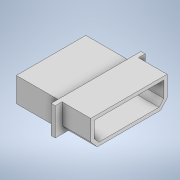
# Autodesk Inventor part: MolexConnector
Saved by Autodesk Inventor 2021 (Build 250183000, 183)
## iProperties
Created: 2021-02-27
Part Number: MolexConnector
Material: Generic
Document SubType Name: Modeling
Designer: Collin
Density: 1 g/cm^3
Appearance: Default
Author: Collin
Autodesk Inventor part; units mm, degrees
ref_plane "YZ Plane" through (0, 0, 0) normal (1, 0, 0) x (0, 1, 0)
ref_plane "XZ Plane" through (0, 0, 0) normal (0, 1, 0) x (-1, 0, 0)
ref_plane "XY Plane" through (0, 0, 0) normal (0, 0, 1) x (1, 0, 0)
sketch "Sketch1" plane through (0, 0, 0) normal (0, 1, 0) x (-1, 0, 0)
  line L0 (-11.8618, -11.6459) -> (11.8618, -11.6459)
  line L1 (11.8618, -11.6459) -> (11.8618, 11.6459)
  line L2 (11.8618, 11.6459) -> (-11.8618, 11.6459)
  line L3 (-11.8618, 11.6459) -> (-11.8618, -11.6459)
  line L4 (-11.8618, -11.6459) -> (11.8618, 11.6459) construction
  line L5 (11.8618, -11.6459) -> (-11.8618, 11.6459) construction
  point P0 (0, 0)
  dimension "d0" = 23.2918
  dimension "d1" = 23.7236
  constraints: 12 end point, 2 midpoint, 2 parallel, 1 horizontal, 1 perpendicular
  measures "d0" distance between parallel lines of L0 L2
  measures "d1" distance of L1.end L2.end
extrude "Extrusion1" add sketch "Sketch1" along normal mid plane 8.509
sketch "Sketch2" plane through (0, 4.2545, 0) normal (0, 1, 0) x (1, 0, 0)
  line L0 (-11.8618, 11.6459) -> (-11.8618, -11.6459) projected
  line L1 (11.8618, 11.6459) -> (-11.8618, 11.6459) projected
  line L2 (-11.8618, -11.6459) -> (1.8542, -11.6459)
  line L3 (1.8542, -11.6459) -> (1.8542, 11.6459)
  line L4 (1.8542, 11.6459) -> (-11.8618, 11.6459)
  line L5 (-11.8618, 11.6459) -> (-11.8618, -11.6459)
  point P0 (0, 0)
  dimension "d4" = 13.716
  constraints: 8 end point, 2 parallel, 1 horizontal, 1 perpendicular, 1 point on line
  measures "d4" distance between parallel lines of L3 L0
extrude "Extrusion2" cut sketch "Sketch2" against normal blind 1.0414
sketch "Sketch3" plane through (0, 3.2131, 0) normal (0, 1, 0) x (1, 0, 0)
  line L0 (-11.8618, -11.6459) -> (-11.8618, 11.6459) projected
  line L1 (1.8542, 11.6459) -> (1.8542, -11.6459) projected
  line L2 (-11.8618, -10.5791) -> (1.8542, -10.5791)
  line L3 (1.8542, -10.5791) -> (1.8542, 10.5791)
  line L4 (1.8542, 10.5791) -> (-11.8618, 10.5791)
  line L5 (-11.8618, 10.5791) -> (-11.8618, -10.5791)
  line L6 (1.8542, -11.6459) -> (-11.8618, -11.6459) projected
  line L7 (-11.8618, 11.6459) -> (1.8542, 11.6459) projected
  line L8 (1.8542, -11.6459) -> (1.8542, -10.5791)
  line L9 (1.8542, 11.6459) -> (1.8542, 10.5791)
  point P0 (0, 0)
  dimension "d7" = 1.0668
  dimension "d8" = 21.1582
  dimension "d9" = 1.0668
  constraints: 12 end point, 2 collinear, 2 parallel, 2 point on line, 1 horizontal, 1 perpendicular
  measures "d7" distance between parallel lines of L6 L2
  measures "d8" distance between parallel lines of L4 L2
  measures "d9" distance between parallel lines of L7 L4
extrude "Extrusion3" cut sketch "Sketch3" against normal up to surface (7.4676 mm away) contours L0 L2 L1 L6 | L0 L7 L1 L4
sketch "Sketch4" plane through (1.8542, 4.2545, -11.6459) normal (-1, 0, 0) x (0, 0, 1)
  line L0 (-2.0701, 0) -> (25.3619, 0)
  line L1 (25.3619, 0) -> (25.3619, -8.509)
  line L2 (25.3619, -8.509) -> (-2.0701, -8.509)
  line L3 (-2.0701, -8.509) -> (-2.0701, 0)
  line L4 (23.2918, -8.509) -> (22.225, -8.509) projected
  line L5 (0, 0) -> (23.2918, 0) projected
  line L6 (23.2918, 0) -> (23.2918, -8.509) projected
  line L7 (0, -8.509) -> (0, 0) projected
  point P0 (11.6459, -4.2545)
  dimension "d12" = 27.432
  dimension "d13" = 2.0701
  dimension "d14" = 2.0701
  constraints: 8 end point, 2 collinear, 2 parallel, 1 horizontal, 1 perpendicular
  measures "d12" distance between parallel lines of L1 L3
  measures "d13" distance between parallel lines of L6 L1
  measures "d14" distance between parallel lines of L3 L7
extrude "Extrusion4" add sketch "Sketch4" against normal blind 1.27 contours L0 L7 L2 L3 | L0 L1 L2 L6
sketch "Sketch5" plane through (11.8618, -4.2545, -11.6459) normal (1, 0, 0) x (0, 0, -1)
  line L0 (-23.2918, 8.509) -> (-23.2918, 0) projected
  line L1 (-23.2918, 2.286) -> (-21.3106, 0)
  line L2 (-21.3106, 0) -> (-1.9812, 0)
  line L3 (0, 0) -> (-23.2918, 0) projected
  line L4 (0, 0) -> (0, 8.509) projected
  line L5 (0, 2.286) -> (-1.9812, 0)
  point P0 (-11.6459, 4.2545)
  dimension "d17" = 19.3294
  dimension "d20" = 6.223
  dimension "d21" = 139.086
  dimension "d22" = 139.086
  constraints: 6 end point, 4 point on line, 1 horizontal alignment
  measures "d17" distance of L1.end L2.end
  measures "d20" distance of L1.start L0.start
  measures "d21" angle of L0 L1
  measures "d22" angle of L4 L5
extrude "Extrusion5" cut sketch "Sketch5" against normal up to surface (8.7376 mm away)
sketch "Sketch6" plane through (11.8618, 4.2545, 11.6459) normal (1, 0, 0) x (0, 0, -1)
  line L0 (21.3106, -8.509) -> (23.2918, -6.223) projected
  line L1 (23.2918, -6.223) -> (23.2918, 0) projected
  line L2 (0, 0) -> (23.2918, 0) projected
  line L3 (0, -6.223) -> (0, 0) projected
  line L4 (0, -6.223) -> (1.9812, -8.509) projected
  line L5 (21.3106, -8.509) -> (1.9812, -8.509) projected
  line L6 (2.4451, -7.493) -> (1.016, -5.844)
  line L7 (1.016, -5.844) -> (1.016, -1.016)
  line L8 (1.016, -1.016) -> (22.2758, -1.016)
  line L9 (22.2758, -1.016) -> (22.2758, -5.844)
  line L10 (22.2758, -5.844) -> (20.8467, -7.493)
  line L11 (20.8467, -7.493) -> (2.4451, -7.493)
  point P0 (11.6459, -4.2545)
  dimension "d25" = 1.016
  constraints: 12 end point, 5 other
  measures "d25" distance between parallel lines of L4 L6
extrude "Extrusion6" cut sketch "Sketch6" against normal up to surface (8.7376 mm away) contours L6 L7 L8 L9 L10 L11
equation "\"d7\" = d9"
equation "\"d13\" = d14"
equation "\"d21\" = d22"
body "Solid1"
